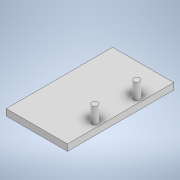
# Autodesk Inventor part: contrabase_fin_carrera
Saved by Autodesk Inventor 2021 (Build 250183000, 183)
## iProperties
Created: 2022-03-27
Part Number: contrabase_fin_carrera
Material: Genérico
Document SubType Name: Modeling
Designer: orgyn
Density: 1 g/cm^3
Appearance: Valor por defecto
Author: orgyn
Autodesk Inventor part; units mm, degrees
ref_plane "YZ Plane" through (0, 0, 0) normal (1, 0, 0) x (0, 1, 0)
ref_plane "XZ Plane" through (0, 0, 0) normal (0, 1, 0) x (-1, 0, 0)
ref_plane "XY Plane" through (0, 0, 0) normal (0, 0, 1) x (1, 0, 0)
sketch "Boceto1" plane through (0, 0, 0) normal (0, 1, 0) x (-1, 0, 0)
  line L0 (0, 0) -> (3, 0)
  line L1 (3, 0) -> (3, -33)
  line L2 (3, -33) -> (0, -33)
  line L3 (0, -33) -> (0, 0)
  dimension "d0" = 3
  dimension "d1" = 33
  constraints: 8 end point, 3 perpendicular, 1 horizontal
  measures "d0" distance of L0.start L0.end
  measures "d1" distance of L0.end L1.end
extrude "Extrusión1" add sketch "Boceto1" along normal blind 2
sketch "Boceto2" plane through (0, 2, 0) normal (0, 1, 0) x (1, 0, 0)
  line L0 (-3, 0) -> (0, 0) projected
  line L1 (-1.5, 0) -> (-1.5, 10)
  line L2 (0, 33) -> (-3, 33) projected
  line L3 (-1.5, 33) -> (-1.5, 23)
  circle A0 centre (-1.5, 10) radius 0.95
  circle A1 centre (-1.5, 23) radius 0.95
  dimension "d4" = 10
  dimension "d5" = 10
  dimension "d8" = 1.9
  dimension "d9" = 1.9
  constraints: 4 end point, 2 centre point, 2 coincident, 2 midpoint, 2 vertical
  measures "d4" distance of L1.start L1.end
  measures "d5" distance of L3.start L3.end
  measures "d8" diameter of A0
  measures "d9" diameter of A1
extrude "Extrusión2" add sketch "Boceto2" along normal blind 5
sketch "Boceto3" plane through (-3, 0, -33) normal (-1, 0, 0) x (0, 0, 1)
  line L0 (0, 0) -> (33, 0) projected
  line L1 (33, 2) -> (0, 2) projected
  line L2 (33, 0) -> (0, 0)
  line L3 (0, 0) -> (0, 2)
  line L4 (0, 2) -> (33, 2)
  line L5 (33, 2) -> (33, 0)
  constraints: 8 end point, 2 parallel, 1 horizontal, 1 perpendicular
extrude "Extrusión3" add sketch "Boceto3" along normal blind 16
